Autodesk Fusion 360 part; units mm, degrees
(part 3 of 7)
  spline S43 degree 5 poles (24.9906, -19.176) (25.0004, -19.1632) (25.0196, -19.1376) (25.0478, -19.0989) (25.084, -19.0467) (25.127, -18.9804) (25.1677, -18.913) (25.2062, -18.8447) (25.2423, -18.7754) (25.276, -18.7052) (25.3074, -18.6343) (25.3364, -18.5627) (25.3629, -18.4906) (25.387, -18.4182) (25.4085, -18.3457) (25.4275, -18.2732) (25.444, -18.2009) (25.4579, -18.1291) (25.4695, -18.0578) (25.4786, -17.9874) (25.4854, -17.9178) (25.4899, -17.8493) (25.4921, -17.7819) (25.4922, -17.7157) (25.4901, -17.6507) (25.486, -17.5872) (25.4801, -17.5253) (25.4725, -17.4654) (25.4635, -17.4079) (25.4532, -17.3532) (25.442, -17.3014) (25.4301, -17.2527) (25.4177, -17.2069) (25.4049, -17.1636) (25.3921, -17.1224) (25.3797, -17.0834) (25.3686, -17.0474) (25.3597, -17.0156) (25.3539, -16.9897) (25.3519, -16.9707) (25.3531, -16.9582) (25.3562, -16.9504) (25.3597, -16.9448) (25.3635, -16.9394) (25.3696, -16.9336) (25.3806, -16.9277) (25.399, -16.9223) (25.4251, -16.9177) (25.4578, -16.9138) (25.4954, -16.9103) (25.5362, -16.9068) (25.5791, -16.9028) (25.624, -16.898) (25.6711, -16.892) (25.7207, -16.8844) (25.7728, -16.875) (25.8273, -16.8635) (25.8839, -16.8498) (25.9421, -16.8339) (26.0015, -16.8157) (26.0618, -16.7951) (26.1226, -16.7722) (26.1837, -16.7468) (26.2451, -16.7189) (26.3067, -16.6886) (26.3684, -16.6557) (26.43, -16.6203) (26.4914, -16.5824) (26.5525, -16.542) (26.6129, -16.4991) (26.6726, -16.4538) (26.7314, -16.4062) (26.7891, -16.3563) (26.8455, -16.3042) (26.9006, -16.25) (26.9541, -16.1938) (27.006, -16.1358) (27.0562, -16.0759) (27.1046, -16.0143) (27.1512, -15.9509) (27.1961, -15.8857) (27.2305, -15.8323) (27.2555, -15.7914) (27.2717, -15.7639) (27.2798, -15.75) knots 0 0 0 0 0 0 0.0125 0.025 0.0375 0.05 0.0625 0.075 0.0875 0.1 0.1125 0.125 0.1375 0.15 0.1625 0.175 0.1875 0.2 0.2125 0.225 0.2375 0.25 0.2625 0.275 0.2875 0.3 0.3125 0.325 0.3375 0.35 0.3625 0.375 0.3875 0.4 0.4125 0.425 0.4375 0.45 0.4625 0.475 0.4875 0.5 0.5125 0.525 0.5375 0.55 0.5625 0.575 0.5875 0.6 0.6125 0.625 0.6375 0.65 0.6625 0.675 0.6875 0.7 0.7125 0.725 0.7375 0.75 0.7625 0.775 0.7875 0.8 0.8125 0.825 0.8375 0.85 0.8625 0.875 0.8875 0.9 0.9125 0.925 0.9375 0.95 0.9625 0.975 0.9875 1 1 1 1 1 1
  spline S44 degree 5 poles (27.2798, -15.75) (27.2878, -15.7361) (27.3035, -15.7082) (27.3264, -15.6661) (27.3555, -15.6096) (27.3895, -15.5382) (27.4211, -15.4662) (27.4502, -15.3934) (27.477, -15.32) (27.5013, -15.246) (27.5232, -15.1716) (27.5426, -15.0968) (27.5594, -15.0219) (27.5738, -14.947) (27.5857, -14.8722) (27.5951, -14.7979) (27.602, -14.7241) (27.6065, -14.651) (27.6086, -14.5789) (27.6085, -14.5078) (27.6061, -14.438) (27.6016, -14.3695) (27.595, -14.3024) (27.5864, -14.2367) (27.5759, -14.1726) (27.5636, -14.1101) (27.5496, -14.0496) (27.5343, -13.9912) (27.5178, -13.9354) (27.5005, -13.8824) (27.4827, -13.8325) (27.4645, -13.7858) (27.4462, -13.742) (27.4278, -13.7007) (27.4098, -13.6616) (27.3924, -13.6246) (27.3767, -13.5903) (27.3637, -13.5599) (27.3546, -13.535) (27.3501, -13.5164) (27.3497, -13.5039) (27.3517, -13.4958) (27.3545, -13.4898) (27.3576, -13.4839) (27.3628, -13.4773) (27.373, -13.47) (27.3905, -13.4623) (27.4158, -13.4543) (27.4477, -13.4462) (27.4846, -13.4378) (27.5245, -13.429) (27.5665, -13.4195) (27.6104, -13.4089) (27.6564, -13.3968) (27.7045, -13.3828) (27.7549, -13.3666) (27.8075, -13.3481) (27.8618, -13.3271) (27.9174, -13.3038) (27.974, -13.278) (28.031, -13.2497) (28.0883, -13.219) (28.1456, -13.1859) (28.2029, -13.1502) (28.26, -13.1121) (28.3168, -13.0715) (28.3733, -13.0283) (28.4292, -12.9827) (28.4845, -12.9347) (28.5388, -12.8843) (28.5921, -12.8316) (28.6442, -12.7767) (28.6948, -12.7196) (28.744, -12.6606) (28.7915, -12.5997) (28.8372, -12.5371) (28.8811, -12.4728) (28.923, -12.4068) (28.963, -12.3394) (29.001, -12.2704) (29.0369, -12.2) (29.064, -12.1426) (29.0835, -12.0988) (29.096, -12.0693) (29.1022, -12.0545) knots 0 0 0 0 0 0 0.0125 0.025 0.0375 0.05 0.0625 0.075 0.0875 0.1 0.1125 0.125 0.1375 0.15 0.1625 0.175 0.1875 0.2 0.2125 0.225 0.2375 0.25 0.2625 0.275 0.2875 0.3 0.3125 0.325 0.3375 0.35 0.3625 0.375 0.3875 0.4 0.4125 0.425 0.4375 0.45 0.4625 0.475 0.4875 0.5 0.5125 0.525 0.5375 0.55 0.5625 0.575 0.5875 0.6 0.6125 0.625 0.6375 0.65 0.6625 0.675 0.6875 0.7 0.7125 0.725 0.7375 0.75 0.7625 0.775 0.7875 0.8 0.8125 0.825 0.8375 0.85 0.8625 0.875 0.8875 0.9 0.9125 0.925 0.9375 0.95 0.9625 0.975 0.9875 1 1 1 1 1 1
  spline S45 degree 5 poles (29.1022, -12.0545) (29.1083, -12.0397) (29.1203, -12.01) (29.1375, -11.9653) (29.159, -11.9055) (29.1833, -11.8303) (29.2052, -11.7547) (29.2246, -11.6787) (29.2416, -11.6024) (29.256, -11.5259) (29.268, -11.4493) (29.2775, -11.3726) (29.2844, -11.2962) (29.2889, -11.22) (29.2909, -11.1444) (29.2905, -11.0694) (29.2877, -10.9953) (29.2826, -10.9223) (29.2753, -10.8505) (29.2659, -10.7801) (29.2545, -10.7112) (29.2411, -10.6438) (29.2258, -10.5781) (29.2087, -10.5142) (29.1899, -10.452) (29.1695, -10.3917) (29.1478, -10.3334) (29.125, -10.2775) (29.1013, -10.2243) (29.0773, -10.1741) (29.0531, -10.127) (29.0289, -10.0831) (29.005, -10.042) (28.9815, -10.0035) (28.9585, -9.967) (28.9365, -9.9326) (28.9164, -9.9006) (28.8995, -9.8722) (28.8873, -9.8487) (28.8804, -9.8308) (28.8783, -9.8185) (28.8793, -9.8102) (28.8813, -9.8039) (28.8835, -9.7977) (28.8879, -9.7905) (28.897, -9.7819) (28.9133, -9.772) (28.9374, -9.7607) (28.968, -9.7485) (29.0034, -9.7354) (29.0418, -9.7214) (29.0823, -9.7065) (29.1244, -9.6903) (29.1684, -9.6723) (29.2143, -9.6521) (29.2622, -9.6295) (29.3118, -9.6043) (29.363, -9.5764) (29.4151, -9.546) (29.4678, -9.513) (29.5206, -9.4776) (29.5734, -9.4397) (29.6259, -9.3993) (29.678, -9.3565) (29.7297, -9.3112) (29.7807, -9.2635) (29.8311, -9.2134) (29.8806, -9.1609) (29.9291, -9.1061) (29.9764, -9.049) (30.0223, -8.9898) (30.0668, -8.9285) (30.1096, -8.8654) (30.1506, -8.8005) (30.1898, -8.7339) (30.2269, -8.6658) (30.262, -8.5963) (30.295, -8.5255) (30.3258, -8.4534) (30.3545, -8.3801) (30.3809, -8.3056) (30.4003, -8.2451) (30.4139, -8.1991) (30.4225, -8.1683) (30.4267, -8.1528) knots 0 0 0 0 0 0 0.0125 0.025 0.0375 0.05 0.0625 0.075 0.0875 0.1 0.1125 0.125 0.1375 0.15 0.1625 0.175 0.1875 0.2 0.2125 0.225 0.2375 0.25 0.2625 0.275 0.2875 0.3 0.3125 0.325 0.3375 0.35 0.3625 0.375 0.3875 0.4 0.4125 0.425 0.4375 0.45 0.4625 0.475 0.4875 0.5 0.5125 0.525 0.5375 0.55 0.5625 0.575 0.5875 0.6 0.6125 0.625 0.6375 0.65 0.6625 0.675 0.6875 0.7 0.7125 0.725 0.7375 0.75 0.7625 0.775 0.7875 0.8 0.8125 0.825 0.8375 0.85 0.8625 0.875 0.8875 0.9 0.9125 0.925 0.9375 0.95 0.9625 0.975 0.9875 1 1 1 1 1 1
  spline S46 degree 5 poles (30.4267, -8.1528) (30.4308, -8.1373) (30.4388, -8.1063) (30.45, -8.0597) (30.4635, -7.9976) (30.4778, -7.9199) (30.4897, -7.8421) (30.499, -7.7642) (30.5058, -7.6864) (30.5102, -7.6086) (30.512, -7.5311) (30.5114, -7.4539) (30.5083, -7.3771) (30.5028, -7.301) (30.495, -7.2258) (30.4848, -7.1515) (30.4723, -7.0785) (30.4578, -7.0067) (30.4412, -6.9365) (30.4226, -6.8679) (30.4023, -6.8011) (30.3802, -6.736) (30.3565, -6.6729) (30.3312, -6.6117) (30.3044, -6.5525) (30.2764, -6.4954) (30.2472, -6.4405) (30.2173, -6.388) (30.1869, -6.3384) (30.1565, -6.2917) (30.1263, -6.2482) (30.0967, -6.2078) (30.0676, -6.1702) (30.0393, -6.135) (30.0117, -6.1019) (29.9854, -6.0706) (29.9613, -6.0416) (29.9409, -6.0156) (29.9256, -5.9939) (29.9165, -5.9771) (29.9129, -5.9651) (29.9127, -5.9568) (29.9139, -5.9502) (29.9153, -5.9438) (29.9186, -5.9361) (29.9265, -5.9264) (29.9415, -5.9144) (29.9638, -5.9001) (29.9926, -5.884) (30.026, -5.8664) (30.0623, -5.8476) (30.1004, -5.8275) (30.1401, -5.8059) (30.1813, -5.7823) (30.2242, -5.7563) (30.2687, -5.7276) (30.3147, -5.6961) (30.3617, -5.6619) (30.4094, -5.6249) (30.4574, -5.5853) (30.5052, -5.5433) (30.5525, -5.4988) (30.5993, -5.4519) (30.6454, -5.4027) (30.6907, -5.3511) (30.7351, -5.2971) (30.7785, -5.2408) (30.8207, -5.1823) (30.8616, -5.1216) (30.9011, -5.0589) (30.9389, -4.9942) (30.975, -4.9277) (31.0092, -4.8595) (31.0414, -4.7897) (31.0715, -4.7186) (31.0994, -4.6463) (31.1252, -4.5728) (31.1486, -4.4983) (31.1698, -4.4228) (31.1886, -4.3463) (31.2051, -4.269) (31.2164, -4.2065) (31.2239, -4.1592) (31.2284, -4.1275) (31.2305, -4.1116) knots 0 0 0 0 0 0 0.0125 0.025 0.0375 0.05 0.0625 0.075 0.0875 0.1 0.1125 0.125 0.1375 0.15 0.1625 0.175 0.1875 0.2 0.2125 0.225 0.2375 0.25 0.2625 0.275 0.2875 0.3 0.3125 0.325 0.3375 0.35 0.3625 0.375 0.3875 0.4 0.4125 0.425 0.4375 0.45 0.4625 0.475 0.4875 0.5 0.5125 0.525 0.5375 0.55 0.5625 0.575 0.5875 0.6 0.6125 0.625 0.6375 0.65 0.6625 0.675 0.6875 0.7 0.7125 0.725 0.7375 0.75 0.7625 0.775 0.7875 0.8 0.8125 0.825 0.8375 0.85 0.8625 0.875 0.8875 0.9 0.9125 0.925 0.9375 0.95 0.9625 0.975 0.9875 1 1 1 1 1 1
  spline S47 degree 5 poles (31.2305, -4.1116) (31.2326, -4.0957) (31.2364, -4.0639) (31.2415, -4.0163) (31.2467, -3.9529) (31.2508, -3.874) (31.2524, -3.7953) (31.2515, -3.7169) (31.2481, -3.6388) (31.2423, -3.5612) (31.234, -3.484) (31.2233, -3.4076) (31.2102, -3.3319) (31.1949, -3.2572) (31.1772, -3.1836) (31.1574, -3.1113) (31.1356, -3.0405) (31.1118, -2.9713) (31.0861, -2.9038) (31.0588, -2.8382) (31.0299, -2.7746) (30.9995, -2.713) (30.9678, -2.6535) (30.9347, -2.5961) (30.9004, -2.5409) (30.8651, -2.4879) (30.8291, -2.4373) (30.7926, -2.3893) (30.756, -2.344) (30.7197, -2.3017) (30.6842, -2.2624) (30.6495, -2.2262) (30.6158, -2.1928) (30.583, -2.1616) (30.5514, -2.1324) (30.5212, -2.1048) (30.4935, -2.0792) (30.4699, -2.0561) (30.452, -2.0365) (30.4407, -2.0211) (30.4356, -2.0097) (30.4343, -2.0014) (30.4346, -1.9948) (30.4352, -1.9882) (30.4375, -1.9801) (30.4441, -1.9695) (30.4573, -1.9557) (30.4776, -1.9386) (30.504, -1.9188) (30.5348, -1.897) (30.5683, -1.8736) (30.6036, -1.8487) (30.6401, -1.8221) (30.6779, -1.7934) (30.717, -1.762) (30.7574, -1.7278) (30.7988, -1.6905) (30.841, -1.6504) (30.8835, -1.6075) (30.9258, -1.5621) (30.9677, -1.5141) (31.0089, -1.4639) (31.0492, -1.4113) (31.0884, -1.3565) (31.1266, -1.2994) (31.1636, -1.2401) (31.1992, -1.1786) (31.2334, -1.1151) (31.2661, -1.0496) (31.297, -0.9822) (31.3261, -0.9131) (31.3532, -0.8424) (31.3782, -0.7704) (31.401, -0.6971) (31.4216, -0.6226) (31.4398, -0.5472) (31.4558, -0.471) (31.4693, -0.3941) (31.4804, -0.3164) (31.4891, -0.2382) (31.4954, -0.1594) (31.4984, -0.0959) (31.4996, -0.0481) (31.5, -0.016) (31.5, 0) knots 0 0 0 0 0 0 0.0125 0.025 0.0375 0.05 0.0625 0.075 0.0875 0.1 0.1125 0.125 0.1375 0.15 0.1625 0.175 0.1875 0.2 0.2125 0.225 0.2375 0.25 0.2625 0.275 0.2875 0.3 0.3125 0.325 0.3375 0.35 0.3625 0.375 0.3875 0.4 0.4125 0.425 0.4375 0.45 0.4625 0.475 0.4875 0.5 0.5125 0.525 0.5375 0.55 0.5625 0.575 0.5875 0.6 0.6125 0.625 0.6375 0.65 0.6625 0.675 0.6875 0.7 0.7125 0.725 0.7375 0.75 0.7625 0.775 0.7875 0.8 0.8125 0.825 0.8375 0.85 0.8625 0.875 0.8875 0.9 0.9125 0.925 0.9375 0.95 0.9625 0.975 0.9875 1 1 1 1 1 1
  spline S48 degree 3 poles (30, 0.0001) (29.9988, 0.2297) (29.9157, 0.4205) (29.8434, 0.5181) (29.8132, 0.5589) (29.7829, 0.5878) (29.7594, 0.6069) (29.7462, 0.6177) (29.7353, 0.6254) (29.6705, 0.6711) (29.63, 0.6997) (29.5735, 0.7321) (29.4481, 0.8468) (29.3588, 0.9283) (29.2058, 1.0812) (29.0859, 1.3313) (28.9916, 1.5279) (28.9531, 1.7366) (28.9425, 1.8414) (28.9328, 1.9377) (28.9245, 2.0161) (28.9468, 2.1921) (28.9748, 2.4126) (29.0852, 2.6848) (29.1806, 2.8335) (29.3575, 3.1091) (29.4389, 3.1467) (29.4891, 3.1933) (29.6004, 3.2968) (29.583, 3.2795) (29.6058, 3.3076) (29.6806, 3.3996) (29.7802, 3.6234) (29.7433, 3.9159) knots 0.001251 0.001251 0.001251 0.001251 0.25 0.25 0.25 0.35404 0.35404 0.35404 0.412746 0.412746 0.412746 0.449449 0.449449 0.449449 0.475576 0.475576 0.475576 0.496118 0.496118 0.496118 0.514995 0.514995 0.514995 0.538647 0.538647 0.538647 0.582499 0.582499 0.582499 0.679826 0.679826 0.679826 0.99875 0.99875 0.99875 0.99875
  spline S49 degree 3 poles (29.7433, 3.9159) (29.7122, 4.1433) (29.6048, 4.3217) (29.5205, 4.409) (29.4852, 4.4455) (29.4514, 4.4703) (29.4256, 4.4861) (29.4111, 4.495) (29.3993, 4.5013) (29.3291, 4.5382) (29.2852, 4.5612) (29.2249, 4.586) (29.0856, 4.6833) (28.9864, 4.7525) (28.8148, 4.8841) (28.6632, 5.1164) (28.5441, 5.299) (28.4788, 5.5009) (28.4546, 5.6034) (28.4323, 5.6976) (28.4139, 5.7743) (28.413, 5.9517) (28.412, 6.1739) (28.4859, 6.4582) (28.5611, 6.6181) (28.7005, 6.9144) (28.7764, 6.9623) (28.82, 7.0151) (28.9168, 7.1322) (28.9019, 7.1128) (28.9208, 7.1436) (28.9829, 7.2446) (29.0525, 7.4795) (28.9777, 7.7647) knots 0.001251 0.001251 0.001251 0.001251 0.25 0.25 0.25 0.35404 0.35404 0.35404 0.412746 0.412746 0.412746 0.449449 0.449449 0.449449 0.475576 0.475576 0.475576 0.496118 0.496118 0.496118 0.514995 0.514995 0.514995 0.538647 0.538647 0.538647 0.582499 0.582499 0.582499 0.679826 0.679826 0.679826 0.99875 0.99875 0.99875 0.99875
  spline S50 degree 3 poles (28.9777, 7.7647) (28.9172, 7.9861) (28.7875, 8.1489) (28.6924, 8.2245) (28.6527, 8.2561) (28.616, 8.2762) (28.5883, 8.2885) (28.5727, 8.2955) (28.5603, 8.3002) (28.4858, 8.3276) (28.4393, 8.3447) (28.3763, 8.3614) (28.2255, 8.4396) (28.1181, 8.4953) (27.9308, 8.6034) (27.7502, 8.8139) (27.6083, 8.9794) (27.5171, 9.1711) (27.4797, 9.2695) (27.4454, 9.36) (27.4171, 9.4336) (27.3931, 9.6094) (27.363, 9.8296) (27.3993, 10.1211) (27.4529, 10.2894) (27.5525, 10.6015) (27.6214, 10.6588) (27.6578, 10.7168) (27.7385, 10.8456) (27.7262, 10.8244) (27.741, 10.8574) (27.7894, 10.9657) (27.8277, 11.2076) (27.7163, 11.4806) knots 0.001251 0.001251 0.001251 0.001251 0.25 0.25 0.25 0.35404 0.35404 0.35404 0.412746 0.412746 0.412746 0.449449 0.449449 0.449449 0.475576 0.475576 0.475576 0.496118 0.496118 0.496118 0.514995 0.514995 0.514995 0.538647 0.538647 0.538647 0.582499 0.582499 0.582499 0.679826 0.679826 0.679826 0.99875 0.99875 0.99875 0.99875
  spline S51 degree 3 poles (27.7163, 11.4806) (27.6274, 11.6922) (27.4775, 11.8368) (27.3735, 11.8992) (27.3299, 11.9254) (27.2909, 11.9405) (27.2619, 11.9492) (27.2455, 11.954) (27.2325, 11.9571) (27.1552, 11.9745) (27.1068, 11.9853) (27.0422, 11.9937) (26.8824, 12.0516) (26.7687, 12.0928) (26.5688, 12.1755) (26.3624, 12.3606) (26.2, 12.5062) (26.0846, 12.6843) (26.0347, 12.7771) (25.9889, 12.8623) (25.9512, 12.9316) (25.9045, 13.1027) (25.8459, 13.3171) (25.8438, 13.6108) (25.875, 13.7847) (25.933, 14.1071) (25.9939, 14.173) (26.0223, 14.2352) (26.0856, 14.3734) (26.0762, 14.3508) (26.0865, 14.3854) (26.1203, 14.4991) (26.1267, 14.744) (25.9807, 15.0001) knots 0.001251 0.001251 0.001251 0.001251 0.25 0.25 0.25 0.35404 0.35404 0.35404 0.412746 0.412746 0.412746 0.449449 0.449449 0.449449 0.475576 0.475576 0.475576 0.496118 0.496118 0.496118 0.514995 0.514995 0.514995 0.538647 0.538647 0.538647 0.582499 0.582499 0.582499 0.679826 0.679826 0.679826 0.99875 0.99875 0.99875 0.99875
  spline S52 degree 3 poles (25.9807, 15.0001) (25.8649, 15.1983) (25.6975, 15.322) (25.5861, 15.3704) (25.5395, 15.3906) (25.4989, 15.4006) (25.469, 15.4053) (25.4521, 15.408) (25.4388, 15.4093) (25.3599, 15.4165) (25.3105, 15.421) (25.2453, 15.4208) (25.0794, 15.4573) (24.9613, 15.4834) (24.7523, 15.5393) (24.5234, 15.6959) (24.3435, 15.819) (24.2058, 15.9805) (24.1443, 16.066) (24.0877, 16.1444) (24.0413, 16.2082) (23.9726, 16.3718) (23.8866, 16.5767) (23.8461, 16.8677) (23.8544, 17.0441) (23.8698, 17.3713) (23.9215, 17.4446) (23.9416, 17.51) (23.9863, 17.6553) (23.9799, 17.6316) (23.9856, 17.6673) (24.0044, 17.7844) (23.9787, 18.028) (23.8005, 18.2629) knots 0.001251 0.001251 0.001251 0.001251 0.25 0.25 0.25 0.35404 0.35404 0.35404 0.412746 0.412746 0.412746 0.449449 0.449449 0.449449 0.475576 0.475576 0.475576 0.496118 0.496118 0.496118 0.514995 0.514995 0.514995 0.538647 0.538647 0.538647 0.582499 0.582499 0.582499 0.679826 0.679826 0.679826 0.99875 0.99875 0.99875 0.99875
  spline S53 degree 3 poles (23.8005, 18.2629) (23.6598, 18.4443) (23.4777, 18.5451) (23.361, 18.5786) (23.3122, 18.5925) (23.2705, 18.5971) (23.2403, 18.5979) (23.2232, 18.5984) (23.2099, 18.5979) (23.1307, 18.5947) (23.0811, 18.5927) (23.0165, 18.5841) (22.8472, 18.5986) (22.7267, 18.609) (22.5123, 18.6372) (22.2649, 18.7625) (22.0704, 18.8611) (21.9129, 19.0033) (21.8407, 19.08) (21.7743, 19.1504) (21.72, 19.2076) (21.6306, 19.3608) (21.5185, 19.5527) (21.4404, 19.8359) (21.4256, 20.012) (21.3981, 20.3383) (21.4399, 20.4177) (21.4513, 20.4852) (21.4766, 20.6351) (21.4734, 20.6108) (21.4744, 20.647) (21.4777, 20.7655) (21.4205, 21.0037) (21.2131, 21.2133) knots 0.001251 0.001251 0.001251 0.001251 0.25 0.25 0.25 0.35404 0.35404 0.35404 0.412746 0.412746 0.412746 0.449449 0.449449 0.449449 0.475576 0.475576 0.475576 0.496118 0.496118 0.496118 0.514995 0.514995 0.514995 0.538647 0.538647 0.538647 0.582499 0.582499 0.582499 0.679826 0.679826 0.679826 0.99875 0.99875 0.99875 0.99875
  spline S54 degree 3 poles (21.2131, 21.2133) (21.05, 21.3747) (20.8562, 21.4509) (20.7361, 21.4688) (20.6859, 21.4763) (20.6441, 21.4754) (20.6139, 21.4722) (20.5969, 21.4705) (20.5838, 21.4683) (20.5057, 21.4548) (20.4568, 21.4463) (20.3939, 21.4293) (20.2242, 21.4217) (20.1033, 21.4162) (19.887, 21.4162) (19.6254, 21.5082) (19.4198, 21.5805) (19.245, 21.701) (19.1634, 21.7675) (19.0884, 21.8287) (19.0271, 21.8783) (18.9184, 22.0185) (18.7823, 22.1942) (18.6679, 22.4648) (18.6302, 22.6374) (18.5604, 22.9574) (18.5914, 23.0415) (18.5939, 23.1099) (18.5994, 23.2618) (18.5994, 23.2373) (18.5957, 23.2733) (18.5835, 23.3912) (18.4957, 23.6199) (18.2627, 23.8007) knots 0.001251 0.001251 0.001251 0.001251 0.25 0.25 0.25 0.35404 0.35404 0.35404 0.412746 0.412746 0.412746 0.449449 0.449449 0.449449 0.475576 0.475576 0.475576 0.496118 0.496118 0.496118 0.514995 0.514995 0.514995 0.538647 0.538647 0.538647 0.582499 0.582499 0.582499 0.679826 0.679826 0.679826 0.99875 0.99875 0.99875 0.99875
  spline S55 degree 3 poles (18.2627, 23.8007) (18.0799, 23.9394) (17.8779, 23.9897) (17.7565, 23.9918) (17.7057, 23.9926) (17.6643, 23.9862) (17.6349, 23.9792) (17.6183, 23.9752) (17.6055, 23.9714) (17.5298, 23.9478) (17.4825, 23.933) (17.4224, 23.908) (17.2551, 23.8782) (17.136, 23.857) (16.9215, 23.8287) (16.6502, 23.8858) (16.4368, 23.9307) (16.2478, 24.0273) (16.1582, 24.0826) (16.0759, 24.1335) (16.0086, 24.1747) (15.8826, 24.2995) (15.7247, 24.4559) (15.576, 24.7092) (15.5161, 24.8754) (15.4051, 25.1836) (15.4249, 25.2711) (15.4184, 25.3392) (15.404, 25.4905) (15.4072, 25.4662) (15.3988, 25.5014) (15.3713, 25.6167) (15.2544, 25.832) (14.9999, 25.9808) knots 0.001251 0.001251 0.001251 0.001251 0.25 0.25 0.25 0.35404 0.35404 0.35404 0.412746 0.412746 0.412746 0.449449 0.449449 0.449449 0.475576 0.475576 0.475576 0.496118 0.496118 0.496118 0.514995 0.514995 0.514995 0.538647 0.538647 0.538647 0.582499 0.582499 0.582499 0.679826 0.679826 0.679826 0.99875 0.99875 0.99875 0.99875
  spline S56 degree 3 poles (14.9999, 25.9808) (14.8005, 26.0945) (14.5936, 26.118) (14.473, 26.1042) (14.4226, 26.0984) (14.3824, 26.0867) (14.3541, 26.0759) (14.3382, 26.0698) (14.326, 26.0643) (14.2541, 26.031) (14.2091, 26.0102) (14.1527, 25.9775) (13.9907, 25.9262) (13.8754, 25.8896) (13.6665, 25.8336) (13.39, 25.8547) (13.1726, 25.8714) (12.9726, 25.9425) (12.8766, 25.9857) (12.7883, 26.0253) (12.7162, 26.0574) (12.575, 26.1647) (12.398, 26.2992) (12.2175, 26.5309) (12.1364, 26.6879) (11.9862, 26.9789) (11.9944, 27.0682) (11.9791, 27.135) (11.9451, 27.2831) (11.9514, 27.2594) (11.9385, 27.2932) (11.8962, 27.4039) (11.7522, 27.6021) (11.4804, 27.7164) knots 0.001251 0.001251 0.001251 0.001251 0.25 0.25 0.25 0.35404 0.35404 0.35404 0.412746 0.412746 0.412746 0.449449 0.449449 0.449449 0.475576 0.475576 0.475576 0.496118 0.496118 0.496118 0.514995 0.514995 0.514995 0.538647 0.538647 0.538647 0.582499 0.582499 0.582499 0.679826 0.679826 0.679826 0.99875 0.99875 0.99875 0.99875
  spline S57 degree 3 poles (11.4804, 27.7164) (11.2679, 27.8031) (11.0597, 27.7994) (10.9419, 27.77) (10.8927, 27.7577) (10.8543, 27.7408) (10.8277, 27.7264) (10.8127, 27.7182) (10.8014, 27.7112) (10.7344, 27.6688) (10.6925, 27.6423) (10.6409, 27.6025) (10.487, 27.5305) (10.3774, 27.4792) (10.1776, 27.3964) (9.9007, 27.3813) (9.683, 27.3694) (9.4754, 27.4138) (9.3746, 27.4441) (9.2819, 27.4719) (9.2063, 27.4943) (9.0522, 27.5822) (8.8592, 27.6924) (8.65, 27.8986) (8.5492, 28.0437) (8.3622, 28.3126) (8.3586, 28.4022) (8.3347, 28.4664) (8.2817, 28.6088) (8.2911, 28.5861) (8.2739, 28.618) (8.2175, 28.7223) (8.0488, 28.8999) (7.7644, 28.9778) knots 0.001251 0.001251 0.001251 0.001251 0.25 0.25 0.25 0.35404 0.35404 0.35404 0.412746 0.412746 0.412746 0.449449 0.449449 0.449449 0.475576 0.475576 0.475576 0.496118 0.496118 0.496118 0.514995 0.514995 0.514995 0.538647 0.538647 0.538647 0.582499 0.582499 0.582499 0.679826 0.679826 0.679826 0.99875 0.99875 0.99875 0.99875
  spline S58 degree 3 poles (7.7644, 28.9778) (7.5424, 29.036) (7.3365, 29.0052) (7.2236, 28.9606) (7.1764, 28.942) (7.1406, 28.9203) (7.1161, 28.9025) (7.1022, 28.8924) (7.0919, 28.884) (7.031, 28.8332) (6.993, 28.8015) (6.947, 28.7553) (6.8038, 28.6638) (6.7019, 28.5987) (6.5146, 28.4905) (6.242, 28.4393) (6.0278, 28.3991) (5.8162, 28.4161) (5.7122, 28.4329) (5.6167, 28.4484) (5.5388, 28.4607) (5.3746, 28.5278) (5.1689, 28.6119) (4.9345, 28.789) (4.8156, 28.9196) (4.5951, 29.1619) (4.5799, 29.2503) (4.5478, 29.3108) (4.4767, 29.445) (4.4889, 29.4238) (4.4677, 29.4531) (4.3982, 29.5491) (4.2078, 29.7033) (3.9157, 29.7434) knots 0.001251 0.001251 0.001251 0.001251 0.25 0.25 0.25 0.35404 0.35404 0.35404 0.412746 0.412746 0.412746 0.449449 0.449449 0.449449 0.475576 0.475576 0.475576 0.496118 0.496118 0.496118 0.514995 0.514995 0.514995 0.538647 0.538647 0.538647 0.582499 0.582499 0.582499 0.679826 0.679826 0.679826 0.99875 0.99875 0.99875 0.99875
  spline S59 degree 3 poles (3.9157, 29.7434) (3.6879, 29.7721) (3.4878, 29.7146) (3.3817, 29.6557) (3.3373, 29.6311) (3.3046, 29.6049) (3.2827, 29.584) (3.2703, 29.5723) (3.2612, 29.5626) (3.2074, 29.5043) (3.1738, 29.4679) (3.1342, 29.4161) (3.0042, 29.3067) (2.9117, 29.2288) (2.7401, 29.097) (2.4766, 29.0108) (2.2694, 28.943) (2.0574, 28.9321) (1.9521, 28.9353) (1.8554, 28.9382) (1.7765, 28.9402) (1.605, 28.9853) (1.39, 29.0418) (1.1346, 29.1868) (0.9996, 29.3008) (0.7494, 29.5122) (0.7228, 29.5978) (0.6831, 29.6536) (0.595, 29.7775) (0.61, 29.758) (0.5851, 29.7843) (0.5036, 29.8704) (0.2947, 29.9984) (-0.0001, 30) knots 0.001251 0.001251 0.001251 0.001251 0.25 0.25 0.25 0.35404 0.35404 0.35404 0.412746 0.412746 0.412746 0.449449 0.449449 0.449449 0.475576 0.475576 0.475576 0.496118 0.496118 0.496118 0.514995 0.514995 0.514995 0.538647 0.538647 0.538647 0.582499 0.582499 0.582499 0.679826 0.679826 0.679826 0.99875 0.99875 0.99875 0.99875
  spline S60 degree 3 poles (-0.0001, 30) (-0.2297, 29.9988) (-0.4205, 29.9157) (-0.5181, 29.8434) (-0.5589, 29.8132) (-0.5878, 29.7829) (-0.6069, 29.7594) (-0.6177, 29.7462) (-0.6254, 29.7353) (-0.6711, 29.6705) (-0.6997, 29.63) (-0.7321, 29.5735) (-0.8468, 29.4481) (-0.9283, 29.3588) (-1.0812, 29.2058) (-1.3313, 29.0859) (-1.5279, 28.9916) (-1.7366, 28.9531) (-1.8414, 28.9425) (-1.9377, 28.9328) (-2.0161, 28.9245) (-2.1921, 28.9468) (-2.4126, 28.9748) (-2.6848, 29.0852) (-2.8335, 29.1806) (-3.1091, 29.3575) (-3.1467, 29.4389) (-3.1933, 29.4891) (-3.2968, 29.6004) (-3.2795, 29.583) (-3.3076, 29.6058) (-3.3996, 29.6806) (-3.6234, 29.7802) (-3.9159, 29.7433) knots 0.001251 0.001251 0.001251 0.001251 0.25 0.25 0.25 0.35404 0.35404 0.35404 0.412746 0.412746 0.412746 0.449449 0.449449 0.449449 0.475576 0.475576 0.475576 0.496118 0.496118 0.496118 0.514995 0.514995 0.514995 0.538647 0.538647 0.538647 0.582499 0.582499 0.582499 0.679826 0.679826 0.679826 0.99875 0.99875 0.99875 0.99875
  spline S61 degree 3 poles (-3.9159, 29.7433) (-4.1433, 29.7122) (-4.3217, 29.6048) (-4.409, 29.5205) (-4.4455, 29.4852) (-4.4703, 29.4514) (-4.4861, 29.4256) (-4.495, 29.4111) (-4.5013, 29.3993) (-4.5382, 29.3291) (-4.5612, 29.2852) (-4.586, 29.2249) (-4.6833, 29.0856) (-4.7525, 28.9864) (-4.8841, 28.8148) (-5.1164, 28.6632) (-5.299, 28.5441) (-5.5009, 28.4788) (-5.6034, 28.4546) (-5.6976, 28.4323) (-5.7743, 28.4139) (-5.9517, 28.413) (-6.1739, 28.412) (-6.4582, 28.4859) (-6.6181, 28.5611) (-6.9144, 28.7005) (-6.9623, 28.7764) (-7.0151, 28.82) (-7.1322, 28.9168) (-7.1128, 28.9019) (-7.1436, 28.9208) (-7.2446, 28.9829) (-7.4795, 29.0525) (-7.7647, 28.9777) knots 0.001251 0.001251 0.001251 0.001251 0.25 0.25 0.25 0.35404 0.35404 0.35404 0.412746 0.412746 0.412746 0.449449 0.449449 0.449449 0.475576 0.475576 0.475576 0.496118 0.496118 0.496118 0.514995 0.514995 0.514995 0.538647 0.538647 0.538647 0.582499 0.582499 0.582499 0.679826 0.679826 0.679826 0.99875 0.99875 0.99875 0.99875
  spline S62 degree 3 poles (-7.7647, 28.9777) (-7.9861, 28.9172) (-8.1489, 28.7875) (-8.2245, 28.6924) (-8.2561, 28.6527) (-8.2762, 28.616) (-8.2885, 28.5883) (-8.2955, 28.5727) (-8.3002, 28.5603) (-8.3276, 28.4858) (-8.3447, 28.4393) (-8.3614, 28.3763) (-8.4396, 28.2255) (-8.4953, 28.1181) (-8.6034, 27.9308) (-8.8139, 27.7502) (-8.9794, 27.6083) (-9.1711, 27.5171) (-9.2695, 27.4797) (-9.36, 27.4454) (-9.4336, 27.4171) (-9.6094, 27.3931) (-9.8296, 27.363) (-10.1211, 27.3993) (-10.2894, 27.4529) (-10.6015, 27.5525) (-10.6588, 27.6214) (-10.7168, 27.6578) (-10.8456, 27.7385) (-10.8244, 27.7262) (-10.8574, 27.741) (-10.9657, 27.7894) (-11.2076, 27.8277) (-11.4806, 27.7163) knots 0.001251 0.001251 0.001251 0.001251 0.25 0.25 0.25 0.35404 0.35404 0.35404 0.412746 0.412746 0.412746 0.449449 0.449449 0.449449 0.475576 0.475576 0.475576 0.496118 0.496118 0.496118 0.514995 0.514995 0.514995 0.538647 0.538647 0.538647 0.582499 0.582499 0.582499 0.679826 0.679826 0.679826 0.99875 0.99875 0.99875 0.99875
  spline S63 degree 3 poles (-11.4806, 27.7163) (-11.6922, 27.6274) (-11.8368, 27.4775) (-11.8992, 27.3735) (-11.9254, 27.3299) (-11.9405, 27.2909) (-11.9492, 27.2619) (-11.954, 27.2455) (-11.9571, 27.2325) (-11.9745, 27.1552) (-11.9853, 27.1068) (-11.9937, 27.0422) (-12.0516, 26.8824) (-12.0928, 26.7687) (-12.1755, 26.5688) (-12.3606, 26.3624) (-12.5062, 26.2) (-12.6843, 26.0846) (-12.7771, 26.0347) (-12.8623, 25.9889) (-12.9316, 25.9512) (-13.1027, 25.9045) (-13.3171, 25.8459) (-13.6108, 25.8438) (-13.7847, 25.875) (-14.1071, 25.933) (-14.173, 25.9939) (-14.2352, 26.0223) (-14.3734, 26.0856) (-14.3508, 26.0762) (-14.3854, 26.0865) (-14.4991, 26.1203) (-14.744, 26.1267) (-15.0001, 25.9807) knots 0.001251 0.001251 0.001251 0.001251 0.25 0.25 0.25 0.35404 0.35404 0.35404 0.412746 0.412746 0.412746 0.449449 0.449449 0.449449 0.475576 0.475576 0.475576 0.496118 0.496118 0.496118 0.514995 0.514995 0.514995 0.538647 0.538647 0.538647 0.582499 0.582499 0.582499 0.679826 0.679826 0.679826 0.99875 0.99875 0.99875 0.99875
  spline S64 degree 3 poles (-15.0001, 25.9807) (-15.1983, 25.8649) (-15.322, 25.6975) (-15.3704, 25.5861) (-15.3906, 25.5395) (-15.4006, 25.4989) (-15.4053, 25.469) (-15.408, 25.4521) (-15.4093, 25.4388) (-15.4165, 25.3599) (-15.421, 25.3105) (-15.4208, 25.2453) (-15.4573, 25.0794) (-15.4834, 24.9613) (-15.5393, 24.7523) (-15.6959, 24.5234) (-15.819, 24.3435) (-15.9805, 24.2058) (-16.066, 24.1443) (-16.1444, 24.0877) (-16.2082, 24.0413) (-16.3718, 23.9726) (-16.5767, 23.8866) (-16.8677, 23.8461) (-17.0441, 23.8544) (-17.3713, 23.8698) (-17.4446, 23.9215) (-17.51, 23.9416) (-17.6553, 23.9863) (-17.6316, 23.9799) (-17.6673, 23.9856) (-17.7844, 24.0044) (-18.028, 23.9787) (-18.2629, 23.8005) knots 0.001251 0.001251 0.001251 0.001251 0.25 0.25 0.25 0.35404 0.35404 0.35404 0.412746 0.412746 0.412746 0.449449 0.449449 0.449449 0.475576 0.475576 0.475576 0.496118 0.496118 0.496118 0.514995 0.514995 0.514995 0.538647 0.538647 0.538647 0.582499 0.582499 0.582499 0.679826 0.679826 0.679826 0.99875 0.99875 0.99875 0.99875
  spline S65 degree 3 poles (-18.2629, 23.8005) (-18.4443, 23.6598) (-18.5451, 23.4777) (-18.5786, 23.361) (-18.5925, 23.3122) (-18.5971, 23.2705) (-18.5979, 23.2403) (-18.5984, 23.2232) (-18.5979, 23.2099) (-18.5947, 23.1307) (-18.5927, 23.0811) (-18.5841, 23.0165) (-18.5986, 22.8472) (-18.609, 22.7267) (-18.6372, 22.5123) (-18.7625, 22.2649) (-18.8611, 22.0704) (-19.0033, 21.9129) (-19.08, 21.8407) (-19.1504, 21.7743) (-19.2076, 21.72) (-19.3608, 21.6306) (-19.5527, 21.5185) (-19.8359, 21.4404) (-20.012, 21.4256) (-20.3383, 21.3981) (-20.4177, 21.4399) (-20.4852, 21.4513) (-20.6351, 21.4766) (-20.6108, 21.4734) (-20.647, 21.4744) (-20.7655, 21.4777) (-21.0037, 21.4205) (-21.2133, 21.2131) knots 0.001251 0.001251 0.001251 0.001251 0.25 0.25 0.25 0.35404 0.35404 0.35404 0.412746 0.412746 0.412746 0.449449 0.449449 0.449449 0.475576 0.475576 0.475576 0.496118 0.496118 0.496118 0.514995 0.514995 0.514995 0.538647 0.538647 0.538647 0.582499 0.582499 0.582499 0.679826 0.679826 0.679826 0.99875 0.99875 0.99875 0.99875
  spline S66 degree 3 poles (-21.2133, 21.2131) (-21.3747, 21.05) (-21.4509, 20.8562) (-21.4688, 20.7361) (-21.4763, 20.6859) (-21.4754, 20.6441) (-21.4722, 20.6139) (-21.4705, 20.5969) (-21.4683, 20.5838) (-21.4548, 20.5057) (-21.4463, 20.4568) (-21.4293, 20.3939) (-21.4217, 20.2242) (-21.4162, 20.1033) (-21.4162, 19.887) (-21.5082, 19.6254) (-21.5805, 19.4198) (-21.701, 19.245) (-21.7675, 19.1634) (-21.8287, 19.0884) (-21.8783, 19.0271) (-22.0185, 18.9184) (-22.1942, 18.7823) (-22.4648, 18.6679) (-22.6374, 18.6302) (-22.9574, 18.5604) (-23.0415, 18.5914) (-23.1099, 18.5939) (-23.2618, 18.5994) (-23.2373, 18.5994) (-23.2733, 18.5957) (-23.3912, 18.5835) (-23.6199, 18.4957) (-23.8007, 18.2627) knots 0.001251 0.001251 0.001251 0.001251 0.25 0.25 0.25 0.35404 0.35404 0.35404 0.412746 0.412746 0.412746 0.449449 0.449449 0.449449 0.475576 0.475576 0.475576 0.496118 0.496118 0.496118 0.514995 0.514995 0.514995 0.538647 0.538647 0.538647 0.582499 0.582499 0.582499 0.679826 0.679826 0.679826 0.99875 0.99875 0.99875 0.99875
  spline S67 degree 3 poles (-23.8007, 18.2627) (-23.9394, 18.0799) (-23.9897, 17.8779) (-23.9918, 17.7565) (-23.9926, 17.7057) (-23.9862, 17.6643) (-23.9792, 17.6349) (-23.9752, 17.6183) (-23.9714, 17.6055) (-23.9478, 17.5298) (-23.933, 17.4825) (-23.908, 17.4224) (-23.8782, 17.2551) (-23.857, 17.136) (-23.8287, 16.9215) (-23.8858, 16.6502) (-23.9307, 16.4368) (-24.0273, 16.2478) (-24.0826, 16.1582) (-24.1335, 16.0759) (-24.1747, 16.0086) (-24.2995, 15.8826) (-24.4559, 15.7247) (-24.7092, 15.576) (-24.8754, 15.5161) (-25.1836, 15.4051) (-25.2711, 15.4249) (-25.3392, 15.4184) (-25.4905, 15.404) (-25.4662, 15.4072) (-25.5014, 15.3988) (-25.6167, 15.3713) (-25.832, 15.2544) (-25.9808, 14.9999) knots 0.001251 0.001251 0.001251 0.001251 0.25 0.25 0.25 0.35404 0.35404 0.35404 0.412746 0.412746 0.412746 0.449449 0.449449 0.449449 0.475576 0.475576 0.475576 0.496118 0.496118 0.496118 0.514995 0.514995 0.514995 0.538647 0.538647 0.538647 0.582499 0.582499 0.582499 0.679826 0.679826 0.679826 0.99875 0.99875 0.99875 0.99875
  spline S68 degree 3 poles (-25.9808, 14.9999) (-26.0945, 14.8005) (-26.118, 14.5936) (-26.1042, 14.473) (-26.0984, 14.4226) (-26.0867, 14.3824) (-26.0759, 14.3541) (-26.0698, 14.3382) (-26.0643, 14.326) (-26.031, 14.2541) (-26.0102, 14.2091) (-25.9775, 14.1527) (-25.9262, 13.9907) (-25.8896, 13.8754) (-25.8336, 13.6665) (-25.8547, 13.39) (-25.8714, 13.1726) (-25.9425, 12.9726) (-25.9857, 12.8766) (-26.0253, 12.7883) (-26.0574, 12.7162) (-26.1647, 12.575) (-26.2992, 12.398) (-26.5309, 12.2175) (-26.6879, 12.1364) (-26.9789, 11.9862) (-27.0682, 11.9944) (-27.135, 11.9791) (-27.2831, 11.9451) (-27.2594, 11.9514) (-27.2932, 11.9385) (-27.4039, 11.8962) (-27.6021, 11.7522) (-27.7164, 11.4804) knots 0.001251 0.001251 0.001251 0.001251 0.25 0.25 0.25 0.35404 0.35404 0.35404 0.412746 0.412746 0.412746 0.449449 0.449449 0.449449 0.475576 0.475576 0.475576 0.496118 0.496118 0.496118 0.514995 0.514995 0.514995 0.538647 0.538647 0.538647 0.582499 0.582499 0.582499 0.679826 0.679826 0.679826 0.99875 0.99875 0.99875 0.99875
  spline S69 degree 3 poles (-27.7164, 11.4804) (-27.8031, 11.2679) (-27.7994, 11.0597) (-27.77, 10.9419) (-27.7577, 10.8927) (-27.7408, 10.8543) (-27.7264, 10.8277) (-27.7182, 10.8127) (-27.7112, 10.8014) (-27.6688, 10.7344) (-27.6423, 10.6925) (-27.6025, 10.6409) (-27.5305, 10.487) (-27.4792, 10.3774) (-27.3964, 10.1776) (-27.3813, 9.9007) (-27.3694, 9.683) (-27.4138, 9.4754) (-27.4441, 9.3746) (-27.4719, 9.2819) (-27.4943, 9.2063) (-27.5822, 9.0522) (-27.6924, 8.8592) (-27.8986, 8.65) (-28.0437, 8.5492) (-28.3126, 8.3622) (-28.4022, 8.3586) (-28.4664, 8.3347) (-28.6088, 8.2817) (-28.5861, 8.2911) (-28.618, 8.2739) (-28.7223, 8.2175) (-28.8999, 8.0488) (-28.9778, 7.7644) knots 0.001251 0.001251 0.001251 0.001251 0.25 0.25 0.25 0.35404 0.35404 0.35404 0.412746 0.412746 0.412746 0.449449 0.449449 0.449449 0.475576 0.475576 0.475576 0.496118 0.496118 0.496118 0.514995 0.514995 0.514995 0.538647 0.538647 0.538647 0.582499 0.582499 0.582499 0.679826 0.679826 0.679826 0.99875 0.99875 0.99875 0.99875
  spline S70 degree 3 poles (-28.9778, 7.7644) (-29.036, 7.5424) (-29.0052, 7.3365) (-28.9606, 7.2236) (-28.942, 7.1764) (-28.9203, 7.1406) (-28.9025, 7.1161) (-28.8924, 7.1022) (-28.884, 7.0919) (-28.8332, 7.031) (-28.8015, 6.993) (-28.7553, 6.947) (-28.6638, 6.8038) (-28.5987, 6.7019) (-28.4905, 6.5146) (-28.4393, 6.242) (-28.3991, 6.0278) (-28.4161, 5.8162) (-28.4329, 5.7122) (-28.4484, 5.6167) (-28.4607, 5.5388) (-28.5278, 5.3746) (-28.6119, 5.1689) (-28.789, 4.9345) (-28.9196, 4.8156) (-29.1619, 4.5951) (-29.2503, 4.5799) (-29.3108, 4.5478) (-29.445, 4.4767) (-29.4238, 4.4889) (-29.4531, 4.4677) (-29.5491, 4.3982) (-29.7033, 4.2078) (-29.7434, 3.9157) knots 0.001251 0.001251 0.001251 0.001251 0.25 0.25 0.25 0.35404 0.35404 0.35404 0.412746 0.412746 0.412746 0.449449 0.449449 0.449449 0.475576 0.475576 0.475576 0.496118 0.496118 0.496118 0.514995 0.514995 0.514995 0.538647 0.538647 0.538647 0.582499 0.582499 0.582499 0.679826 0.679826 0.679826 0.99875 0.99875 0.99875 0.99875
  spline S71 degree 3 poles (-29.7434, 3.9157) (-29.7721, 3.6879) (-29.7146, 3.4878) (-29.6557, 3.3817) (-29.6311, 3.3373) (-29.6049, 3.3046) (-29.584, 3.2827) (-29.5723, 3.2703) (-29.5626, 3.2612) (-29.5043, 3.2074) (-29.4679, 3.1738) (-29.4161, 3.1342) (-29.3067, 3.0042) (-29.2288, 2.9117) (-29.097, 2.7401) (-29.0108, 2.4766) (-28.943, 2.2694) (-28.9321, 2.0574) (-28.9353, 1.9521) (-28.9382, 1.8554) (-28.9402, 1.7765) (-28.9853, 1.605) (-29.0418, 1.39) (-29.1868, 1.1346) (-29.3008, 0.9996) (-29.5122, 0.7494) (-29.5978, 0.7228) (-29.6536, 0.6831) (-29.7775, 0.595) (-29.758, 0.61) (-29.7843, 0.5851) (-29.8704, 0.5036) (-29.9984, 0.2947) (-30, -0.0001) knots 0.001251 0.001251 0.001251 0.001251 0.25 0.25 0.25 0.35404 0.35404 0.35404 0.412746 0.412746 0.412746 0.449449 0.449449 0.449449 0.475576 0.475576 0.475576 0.496118 0.496118 0.496118 0.514995 0.514995 0.514995 0.538647 0.538647 0.538647 0.582499 0.582499 0.582499 0.679826 0.679826 0.679826 0.99875 0.99875 0.99875 0.99875
  spline S72 degree 3 poles (-30, -0.0001) (-29.9988, -0.2297) (-29.9157, -0.4205) (-29.8434, -0.5181) (-29.8132, -0.5589) (-29.7829, -0.5878) (-29.7594, -0.6069) (-29.7462, -0.6177) (-29.7353, -0.6254) (-29.6705, -0.6711) (-29.63, -0.6997) (-29.5735, -0.7321) (-29.4481, -0.8468) (-29.3588, -0.9283) (-29.2058, -1.0812) (-29.0859, -1.3313) (-28.9916, -1.5279) (-28.9531, -1.7366) (-28.9425, -1.8414) (-28.9328, -1.9377) (-28.9245, -2.0161) (-28.9468, -2.1921) (-28.9748, -2.4126) (-29.0852, -2.6848) (-29.1806, -2.8335) (-29.3575, -3.1091) (-29.4389, -3.1467) (-29.4891, -3.1933) (-29.6004, -3.2968) (-29.583, -3.2795) (-29.6058, -3.3076) (-29.6806, -3.3996) (-29.7802, -3.6234) (-29.7433, -3.9159) knots 0.001251 0.001251 0.001251 0.001251 0.25 0.25 0.25 0.35404 0.35404 0.35404 0.412746 0.412746 0.412746 0.449449 0.449449 0.449449 0.475576 0.475576 0.475576 0.496118 0.496118 0.496118 0.514995 0.514995 0.514995 0.538647 0.538647 0.538647 0.582499 0.582499 0.582499 0.679826 0.679826 0.679826 0.99875 0.99875 0.99875 0.99875
  spline S73 degree 3 poles (-29.7433, -3.9159) (-29.7122, -4.1433) (-29.6048, -4.3217) (-29.5205, -4.409) (-29.4852, -4.4455) (-29.4514, -4.4703) (-29.4256, -4.4861) (-29.4111, -4.495) (-29.3993, -4.5013) (-29.3291, -4.5382) (-29.2852, -4.5612) (-29.2249, -4.586) (-29.0856, -4.6833) (-28.9864, -4.7525) (-28.8148, -4.8841) (-28.6632, -5.1164) (-28.5441, -5.299) (-28.4788, -5.5009) (-28.4546, -5.6034) (-28.4323, -5.6976) (-28.4139, -5.7743) (-28.413, -5.9517) (-28.412, -6.1739) (-28.4859, -6.4582) (-28.5611, -6.6181) (-28.7005, -6.9144) (-28.7764, -6.9623) (-28.82, -7.0151) (-28.9168, -7.1322) (-28.9019, -7.1128) (-28.9208, -7.1436) (-28.9829, -7.2446) (-29.0525, -7.4795) (-28.9777, -7.7647) knots 0.001251 0.001251 0.001251 0.001251 0.25 0.25 0.25 0.35404 0.35404 0.35404 0.412746 0.412746 0.412746 0.449449 0.449449 0.449449 0.475576 0.475576 0.475576 0.496118 0.496118 0.496118 0.514995 0.514995 0.514995 0.538647 0.538647 0.538647 0.582499 0.582499 0.582499 0.679826 0.679826 0.679826 0.99875 0.99875 0.99875 0.99875
  spline S74 degree 3 poles (-28.9777, -7.7647) (-28.9172, -7.9861) (-28.7875, -8.1489) (-28.6924, -8.2245) (-28.6527, -8.2561) (-28.616, -8.2762) (-28.5883, -8.2885) (-28.5727, -8.2955) (-28.5603, -8.3002) (-28.4858, -8.3276) (-28.4393, -8.3447) (-28.3763, -8.3614) (-28.2255, -8.4396) (-28.1181, -8.4953) (-27.9308, -8.6034) (-27.7502, -8.8139) (-27.6083, -8.9794) (-27.5171, -9.1711) (-27.4797, -9.2695) (-27.4454, -9.36) (-27.4171, -9.4336) (-27.3931, -9.6094) (-27.363, -9.8296) (-27.3993, -10.1211) (-27.4529, -10.2894) (-27.5525, -10.6015) (-27.6214, -10.6588) (-27.6578, -10.7168) (-27.7385, -10.8456) (-27.7262, -10.8244) (-27.741, -10.8574) (-27.7894, -10.9657) (-27.8277, -11.2076) (-27.7163, -11.4806) knots 0.001251 0.001251 0.001251 0.001251 0.25 0.25 0.25 0.35404 0.35404 0.35404 0.412746 0.412746 0.412746 0.449449 0.449449 0.449449 0.475576 0.475576 0.475576 0.496118 0.496118 0.496118 0.514995 0.514995 0.514995 0.538647 0.538647 0.538647 0.582499 0.582499 0.582499 0.679826 0.679826 0.679826 0.99875 0.99875 0.99875 0.99875
  spline S75 degree 3 poles (-27.7163, -11.4806) (-27.6274, -11.6922) (-27.4775, -11.8368) (-27.3735, -11.8992) (-27.3299, -11.9254) (-27.2909, -11.9405) (-27.2619, -11.9492) (-27.2455, -11.954) (-27.2325, -11.9571) (-27.1552, -11.9745) (-27.1068, -11.9853) (-27.0422, -11.9937) (-26.8824, -12.0516) (-26.7687, -12.0928) (-26.5688, -12.1755) (-26.3624, -12.3606) (-26.2, -12.5062) (-26.0846, -12.6843) (-26.0347, -12.7771) (-25.9889, -12.8623) (-25.9512, -12.9316) (-25.9045, -13.1027) (-25.8459, -13.3171) (-25.8438, -13.6108) (-25.875, -13.7847) (-25.933, -14.1071) (-25.9939, -14.173) (-26.0223, -14.2352) (-26.0856, -14.3734) (-26.0762, -14.3508) (-26.0865, -14.3854) (-26.1203, -14.4991) (-26.1267, -14.744) (-25.9807, -15.0001) knots 0.001251 0.001251 0.001251 0.001251 0.25 0.25 0.25 0.35404 0.35404 0.35404 0.412746 0.412746 0.412746 0.449449 0.449449 0.449449 0.475576 0.475576 0.475576 0.496118 0.496118 0.496118 0.514995 0.514995 0.514995 0.538647 0.538647 0.538647 0.582499 0.582499 0.582499 0.679826 0.679826 0.679826 0.99875 0.99875 0.99875 0.99875
  spline S76 degree 3 poles (-25.9807, -15.0001) (-25.8649, -15.1983) (-25.6975, -15.322) (-25.5861, -15.3704) (-25.5395, -15.3906) (-25.4989, -15.4006) (-25.469, -15.4053) (-25.4521, -15.408) (-25.4388, -15.4093) (-25.3599, -15.4165) (-25.3105, -15.421) (-25.2453, -15.4208) (-25.0794, -15.4573) (-24.9613, -15.4834) (-24.7523, -15.5393) (-24.5234, -15.6959) (-24.3435, -15.819) (-24.2058, -15.9805) (-24.1443, -16.066) (-24.0877, -16.1444) (-24.0413, -16.2082) (-23.9726, -16.3718) (-23.8866, -16.5767) (-23.8461, -16.8677) (-23.8544, -17.0441) (-23.8698, -17.3713) (-23.9215, -17.4446) (-23.9416, -17.51) (-23.9863, -17.6553) (-23.9799, -17.6316) (-23.9856, -17.6673) (-24.0044, -17.7844) (-23.9787, -18.028) (-23.8005, -18.2629) knots 0.001251 0.001251 0.001251 0.001251 0.25 0.25 0.25 0.35404 0.35404 0.35404 0.412746 0.412746 0.412746 0.449449 0.449449 0.449449 0.475576 0.475576 0.475576 0.496118 0.496118 0.496118 0.514995 0.514995 0.514995 0.538647 0.538647 0.538647 0.582499 0.582499 0.582499 0.679826 0.679826 0.679826 0.99875 0.99875 0.99875 0.99875
  spline S77 degree 3 poles (-23.8005, -18.2629) (-23.6598, -18.4443) (-23.4777, -18.5451) (-23.361, -18.5786) (-23.3122, -18.5925) (-23.2705, -18.5971) (-23.2403, -18.5979) (-23.2232, -18.5984) (-23.2099, -18.5979) (-23.1307, -18.5947) (-23.0811, -18.5927) (-23.0165, -18.5841) (-22.8472, -18.5986) (-22.7267, -18.609) (-22.5123, -18.6372) (-22.2649, -18.7625) (-22.0704, -18.8611) (-21.9129, -19.0033) (-21.8407, -19.08) (-21.7743, -19.1504) (-21.72, -19.2076) (-21.6306, -19.3608) (-21.5185, -19.5527) (-21.4404, -19.8359) (-21.4256, -20.012) (-21.3981, -20.3383) (-21.4399, -20.4177) (-21.4513, -20.4852) (-21.4766, -20.6351) (-21.4734, -20.6108) (-21.4744, -20.647) (-21.4777, -20.7655) (-21.4205, -21.0037) (-21.2131, -21.2133) knots 0.001251 0.001251 0.001251 0.001251 0.25 0.25 0.25 0.35404 0.35404 0.35404 0.412746 0.412746 0.412746 0.449449 0.449449 0.449449 0.475576 0.475576 0.475576 0.496118 0.496118 0.496118 0.514995 0.514995 0.514995 0.538647 0.538647 0.538647 0.582499 0.582499 0.582499 0.679826 0.679826 0.679826 0.99875 0.99875 0.99875 0.99875
  spline S78 degree 3 poles (-21.2131, -21.2133) (-21.05, -21.3747) (-20.8562, -21.4509) (-20.7361, -21.4688) (-20.6859, -21.4763) (-20.6441, -21.4754) (-20.6139, -21.4722) (-20.5969, -21.4705) (-20.5838, -21.4683) (-20.5057, -21.4548) (-20.4568, -21.4463) (-20.3939, -21.4293) (-20.2242, -21.4217) (-20.1033, -21.4162) (-19.887, -21.4162) (-19.6254, -21.5082) (-19.4198, -21.5805) (-19.245, -21.701) (-19.1634, -21.7675) (-19.0884, -21.8287) (-19.0271, -21.8783) (-18.9184, -22.0185) (-18.7823, -22.1942) (-18.6679, -22.4648) (-18.6302, -22.6374) (-18.5604, -22.9574) (-18.5914, -23.0415) (-18.5939, -23.1099) (-18.5994, -23.2618) (-18.5994, -23.2373) (-18.5957, -23.2733) (-18.5835, -23.3912) (-18.4957, -23.6199) (-18.2627, -23.8007) knots 0.001251 0.001251 0.001251 0.001251 0.25 0.25 0.25 0.35404 0.35404 0.35404 0.412746 0.412746 0.412746 0.449449 0.449449 0.449449 0.475576 0.475576 0.475576 0.496118 0.496118 0.496118 0.514995 0.514995 0.514995 0.538647 0.538647 0.538647 0.582499 0.582499 0.582499 0.679826 0.679826 0.679826 0.99875 0.99875 0.99875 0.99875
  spline S79 degree 3 poles (-18.2627, -23.8007) (-18.0799, -23.9394) (-17.8779, -23.9897) (-17.7565, -23.9918) (-17.7057, -23.9926) (-17.6643, -23.9862) (-17.6349, -23.9792) (-17.6183, -23.9752) (-17.6055, -23.9714) (-17.5298, -23.9478) (-17.4825, -23.933) (-17.4224, -23.908) (-17.2551, -23.8782) (-17.136, -23.857) (-16.9215, -23.8287) (-16.6502, -23.8858) (-16.4368, -23.9307) (-16.2478, -24.0273) (-16.1582, -24.0826) (-16.0759, -24.1335) (-16.0086, -24.1747) (-15.8826, -24.2995) (-15.7247, -24.4559) (-15.576, -24.7092) (-15.5161, -24.8754) (-15.4051, -25.1836) (-15.4249, -25.2711) (-15.4184, -25.3392) (-15.404, -25.4905) (-15.4072, -25.4662) (-15.3988, -25.5014) (-15.3713, -25.6167) (-15.2544, -25.832) (-14.9999, -25.9808) knots 0.001251 0.001251 0.001251 0.001251 0.25 0.25 0.25 0.35404 0.35404 0.35404 0.412746 0.412746 0.412746 0.449449 0.449449 0.449449 0.475576 0.475576 0.475576 0.496118 0.496118 0.496118 0.514995 0.514995 0.514995 0.538647 0.538647 0.538647 0.582499 0.582499 0.582499 0.679826 0.679826 0.679826 0.99875 0.99875 0.99875 0.99875
  spline S80 degree 3 poles (-14.9999, -25.9808) (-14.8005, -26.0945) (-14.5936, -26.118) (-14.473, -26.1042) (-14.4226, -26.0984) (-14.3824, -26.0867) (-14.3541, -26.0759) (-14.3382, -26.0698) (-14.326, -26.0643) (-14.2541, -26.031) (-14.2091, -26.0102) (-14.1527, -25.9775) (-13.9907, -25.9262) (-13.8754, -25.8896) (-13.6665, -25.8336) (-13.39, -25.8547) (-13.1726, -25.8714) (-12.9726, -25.9425) (-12.8766, -25.9857) (-12.7883, -26.0253) (-12.7162, -26.0574) (-12.575, -26.1647) (-12.398, -26.2992) (-12.2175, -26.5309) (-12.1364, -26.6879) (-11.9862, -26.9789) (-11.9944, -27.0682) (-11.9791, -27.135) (-11.9451, -27.2831) (-11.9514, -27.2594) (-11.9385, -27.2932) (-11.8962, -27.4039) (-11.7522, -27.6021) (-11.4804, -27.7164) knots 0.001251 0.001251 0.001251 0.001251 0.25 0.25 0.25 0.35404 0.35404 0.35404 0.412746 0.412746 0.412746 0.449449 0.449449 0.449449 0.475576 0.475576 0.475576 0.496118 0.496118 0.496118 0.514995 0.514995 0.514995 0.538647 0.538647 0.538647 0.582499 0.582499 0.582499 0.679826 0.679826 0.679826 0.99875 0.99875 0.99875 0.99875
  spline S81 degree 3 poles (-11.4804, -27.7164) (-11.2679, -27.8031) (-11.0597, -27.7994) (-10.9419, -27.77) (-10.8927, -27.7577) (-10.8543, -27.7408) (-10.8277, -27.7264) (-10.8127, -27.7182) (-10.8014, -27.7112) (-10.7344, -27.6688) (-10.6925, -27.6423) (-10.6409, -27.6025) (-10.487, -27.5305) (-10.3774, -27.4792) (-10.1776, -27.3964) (-9.9007, -27.3813) (-9.683, -27.3694) (-9.4754, -27.4138) (-9.3746, -27.4441) (-9.2819, -27.4719) (-9.2063, -27.4943) (-9.0522, -27.5822) (-8.8592, -27.6924) (-8.65, -27.8986) (-8.5492, -28.0437) (-8.3622, -28.3126) (-8.3586, -28.4022) (-8.3347, -28.4664) (-8.2817, -28.6088) (-8.2911, -28.5861) (-8.2739, -28.618) (-8.2175, -28.7223) (-8.0488, -28.8999) (-7.7644, -28.9778) knots 0.001251 0.001251 0.001251 0.001251 0.25 0.25 0.25 0.35404 0.35404 0.35404 0.412746 0.412746 0.412746 0.449449 0.449449 0.449449 0.475576 0.475576 0.475576 0.496118 0.496118 0.496118 0.514995 0.514995 0.514995 0.538647 0.538647 0.538647 0.582499 0.582499 0.582499 0.679826 0.679826 0.679826 0.99875 0.99875 0.99875 0.99875
  spline S82 degree 3 poles (-7.7644, -28.9778) (-7.5424, -29.036) (-7.3365, -29.0052) (-7.2236, -28.9606) (-7.1764, -28.942) (-7.1406, -28.9203) (-7.1161, -28.9025) (-7.1022, -28.8924) (-7.0919, -28.884) (-7.031, -28.8332) (-6.993, -28.8015) (-6.947, -28.7553) (-6.8038, -28.6638) (-6.7019, -28.5987) (-6.5146, -28.4905) (-6.242, -28.4393) (-6.0278, -28.3991) (-5.8162, -28.4161) (-5.7122, -28.4329) (-5.6167, -28.4484) (-5.5388, -28.4607) (-5.3746, -28.5278) (-5.1689, -28.6119) (-4.9345, -28.789) (-4.8156, -28.9196) (-4.5951, -29.1619) (-4.5799, -29.2503) (-4.5478, -29.3108) (-4.4767, -29.445) (-4.4889, -29.4238) (-4.4677, -29.4531) (-4.3982, -29.5491) (-4.2078, -29.7033) (-3.9157, -29.7434) knots 0.001251 0.001251 0.001251 0.001251 0.25 0.25 0.25 0.35404 0.35404 0.35404 0.412746 0.412746 0.412746 0.449449 0.449449 0.449449 0.475576 0.475576 0.475576 0.496118 0.496118 0.496118 0.514995 0.514995 0.514995 0.538647 0.538647 0.538647 0.582499 0.582499 0.582499 0.679826 0.679826 0.679826 0.99875 0.99875 0.99875 0.99875
  spline S83 degree 3 poles (-3.9157, -29.7434) (-3.6879, -29.7721) (-3.4878, -29.7146) (-3.3817, -29.6557) (-3.3373, -29.6311) (-3.3046, -29.6049) (-3.2827, -29.584) (-3.2703, -29.5723) (-3.2612, -29.5626) (-3.2074, -29.5043) (-3.1738, -29.4679) (-3.1342, -29.4161) (-3.0042, -29.3067) (-2.9117, -29.2288) (-2.7401, -29.097) (-2.4766, -29.0108) (-2.2694, -28.943) (-2.0574, -28.9321) (-1.9521, -28.9353) (-1.8554, -28.9382) (-1.7765, -28.9402) (-1.605, -28.9853) (-1.39, -29.0418) (-1.1346, -29.1868) (-0.9996, -29.3008) (-0.7494, -29.5122) (-0.7228, -29.5978) (-0.6831, -29.6536) (-0.595, -29.7775) (-0.61, -29.758) (-0.5851, -29.7843) (-0.5036, -29.8704) (-0.2947, -29.9984) (0.0001, -30) knots 0.001251 0.001251 0.001251 0.001251 0.25 0.25 0.25 0.35404 0.35404 0.35404 0.412746 0.412746 0.412746 0.449449 0.449449 0.449449 0.475576 0.475576 0.475576 0.496118 0.496118 0.496118 0.514995 0.514995 0.514995 0.538647 0.538647 0.538647 0.582499 0.582499 0.582499 0.679826 0.679826 0.679826 0.99875 0.99875 0.99875 0.99875
  spline S84 degree 3 poles (0.0001, -30) (0.2297, -29.9988) (0.4205, -29.9157) (0.5181, -29.8434) (0.5589, -29.8132) (0.5878, -29.7829) (0.6069, -29.7594) (0.6177, -29.7462) (0.6254, -29.7353) (0.6711, -29.6705) (0.6997, -29.63) (0.7321, -29.5735) (0.8468, -29.4481) (0.9283, -29.3588) (1.0812, -29.2058) (1.3313, -29.0859) (1.5279, -28.9916) (1.7366, -28.9531) (1.8414, -28.9425) (1.9377, -28.9328) (2.0161, -28.9245) (2.1921, -28.9468) (2.4126, -28.9748) (2.6848, -29.0852) (2.8335, -29.1806) (3.1091, -29.3575) (3.1467, -29.4389) (3.1933, -29.4891) (3.2968, -29.6004) (3.2795, -29.583) (3.3076, -29.6058) (3.3996, -29.6806) (3.6234, -29.7802) (3.9159, -29.7433) knots 0.001251 0.001251 0.001251 0.001251 0.25 0.25 0.25 0.35404 0.35404 0.35404 0.412746 0.412746 0.412746 0.449449 0.449449 0.449449 0.475576 0.475576 0.475576 0.496118 0.496118 0.496118 0.514995 0.514995 0.514995 0.538647 0.538647 0.538647 0.582499 0.582499 0.582499 0.679826 0.679826 0.679826 0.99875 0.99875 0.99875 0.99875
  spline S85 degree 3 poles (3.9159, -29.7433) (4.1433, -29.7122) (4.3217, -29.6048) (4.409, -29.5205) (4.4455, -29.4852) (4.4703, -29.4514) (4.4861, -29.4256) (4.495, -29.4111) (4.5013, -29.3993) (4.5382, -29.3291) (4.5612, -29.2852) (4.586, -29.2249) (4.6833, -29.0856) (4.7525, -28.9864) (4.8841, -28.8148) (5.1164, -28.6632) (5.299, -28.5441) (5.5009, -28.4788) (5.6034, -28.4546) (5.6976, -28.4323) (5.7743, -28.4139) (5.9517, -28.413) (6.1739, -28.412) (6.4582, -28.4859) (6.6181, -28.5611) (6.9144, -28.7005) (6.9623, -28.7764) (7.0151, -28.82) (7.1322, -28.9168) (7.1128, -28.9019) (7.1436, -28.9208) (7.2446, -28.9829) (7.4795, -29.0525) (7.7647, -28.9777) knots 0.001251 0.001251 0.001251 0.001251 0.25 0.25 0.25 0.35404 0.35404 0.35404 0.412746 0.412746 0.412746 0.449449 0.449449 0.449449 0.475576 0.475576 0.475576 0.496118 0.496118 0.496118 0.514995 0.514995 0.514995 0.538647 0.538647 0.538647 0.582499 0.582499 0.582499 0.679826 0.679826 0.679826 0.99875 0.99875 0.99875 0.99875